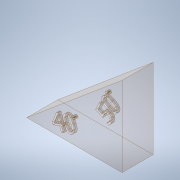
# Autodesk Inventor part: 40-50-4in-Template
Saved by Autodesk Inventor 2020.2 (Build 242310000, 310)
## iProperties
Created: 2020-01-27
Part Number: 40-50-4in-Template
Material: PET Plastic
Document SubType Name: Modeling
Designer: robst
Density: 1.541 g/cm^3
Appearance: Polycarbonate - Smoked
Author: robst
Autodesk Inventor part; units mm, degrees
ref_plane "YZ Plane" through (0, 0, 0) normal (1, 0, 0) x (0, 1, 0)
ref_plane "XZ Plane" through (0, 0, 0) normal (0, 1, 0) x (-1, 0, 0)
ref_plane "XY Plane" through (0, 0, 0) normal (0, 0, 1) x (1, 0, 0)
sketch "Sketch1" plane through (0, 0, 0) normal (0, 0, 1) x (1, 0, 0)
  line L0 (0, 0) -> (77.8301, 65.3072)
  line L1 (0, 0) -> (101.6, 0) construction
  line L2 (77.8301, 65.3072) -> (77.8301, 0)
  line L3 (77.8301, 0) -> (0, 0)
  dimension "d0" = 101.6
  dimension "d1" = 40
  constraints: 8 end point, 1 equal length, 1 horizontal, 1 perpendicular, 1 vertical
  measures "d0" distance of L0.start L0.end
  measures "d1" angle of L1 L0
extrude "Extrusion1" add sketch "Sketch1" along normal mid plane 25.4
sketch "Sketch2" plane through (0, 0, 12.7) normal (0, 0, 1) x (1, 0, 0)
  line L0 (0, 0) -> (77.8301, 0) construction
  line L1 (0, 0) -> (77.8301, 28.3278) construction
  line L2 (77.8301, 0) -> (77.8301, 65.3072) construction
  line L3 (29.7312, 8.7075) -> (28.3096, 8.1901)
  line L4 (28.3096, 8.1901) -> (29.8021, 4.0895)
  line L5 (29.8021, 4.0895) -> (28.2644, 3.5299)
  line L6 (28.2644, 3.5299) -> (26.7719, 7.6304)
  line L7 (26.7719, 7.6304) -> (21.5012, 5.712)
  line L8 (21.5012, 5.712) -> (20.8887, 7.3948)
  line L9 (20.8887, 7.3948) -> (23.9884, 15.4886)
  line L10 (23.9884, 15.4886) -> (25.4584, 16.0236)
  line L11 (25.4584, 16.0236) -> (27.8414, 9.4763)
  line L12 (27.8414, 9.4763) -> (29.2631, 9.9938)
  line L13 (29.2631, 9.9938) -> (29.7312, 8.7075)
  line L14 (26.3037, 8.9166) -> (24.6071, 13.5781)
  line L15 (24.6071, 13.5781) -> (22.2902, 7.4559)
  line L16 (22.2902, 7.4559) -> (26.3037, 8.9166)
  spline S0 degree 2 poles (37.7558, 13.742) (38.9245, 10.5312) (38.1527, 6.8442) (36.2088, 6.1366) knots 0 0 0 1 2 2 2
  spline S1 degree 2 poles (36.2088, 6.1366) (34.2359, 5.4186) (31.2729, 7.812) (30.1289, 10.9551) knots 0 0 0 1 2 2 2
  spline S2 degree 2 poles (30.1289, 10.9551) (28.9532, 14.1852) (29.7321, 17.8529) (31.6856, 18.564) knots 0 0 0 1 2 2 2
  spline S3 degree 2 poles (31.6856, 18.564) (33.6488, 19.2785) (36.6224, 16.8561) (37.7558, 13.742) knots 0 0 0 1 2 2 2
  spline S4 degree 2 poles (37.0291, 9.3594) (37.0465, 10.0339) (36.5781, 11.9224) (36.1311, 13.1506) knots 0 0 0 1 2 2 2
  spline S5 degree 2 poles (36.1311, 13.1506) (35.6841, 14.3789) (34.8324, 16.117) (34.3689, 16.6382) knots 0 0 0 1 2 2 2
  spline S6 degree 2 poles (34.3689, 16.6382) (33.9053, 17.1595) (32.8352, 17.4819) (32.1679, 17.239) knots 0 0 0 1 2 2 2
  spline S7 degree 2 poles (32.1679, 17.239) (31.5005, 16.9961) (30.8686, 16.0542) (30.846, 15.3341) knots 0 0 0 1 2 2 2
  spline S8 degree 2 poles (30.846, 15.3341) (30.826, 14.6368) (31.3277, 12.7166) (31.7536, 11.5464) knots 0 0 0 1 2 2 2
  spline S9 degree 2 poles (31.7536, 11.5464) (32.2112, 10.2892) (32.9784, 8.6627) (33.4692, 8.0966) knots 0 0 0 1 2 2 2
  spline S10 degree 2 poles (33.4692, 8.0966) (33.9266, 7.5622) (35.0302, 7.2081) (35.7266, 7.4616) knots 0 0 0 1 2 2 2
  spline S11 degree 2 poles (35.7266, 7.4616) (36.3842, 7.7009) (37.0161, 8.6428) (37.0291, 9.3594) knots 0 0 0 1 2 2 2
  spline S12 degree 2 poles (38.4763, 17.6439) (37.9694, 17.4594) (36.9953, 17.9137) (36.815, 18.409) knots 0 0 0 1 2 2 2
  spline S13 degree 2 poles (36.815, 18.409) (36.6305, 18.9159) (37.0848, 19.89) (37.5916, 20.0745) knots 0 0 0 1 2 2 2
  spline S14 degree 2 poles (37.5916, 20.0745) (38.087, 20.2548) (39.0611, 19.8005) (39.2456, 19.2937) knots 0 0 0 1 2 2 2
  spline S15 degree 2 poles (39.2456, 19.2937) (39.4259, 18.7983) (38.9716, 17.8242) (38.4763, 17.6439) knots 0 0 0 1 2 2 2
  spline S16 degree 2 poles (37.9564, 19.0723) (37.7375, 18.9926) (37.8172, 18.7738) knots 0 0 0 1 1 1
  spline S17 degree 2 poles (37.8172, 18.7738) (37.8926, 18.5664) (38.1115, 18.6461) knots 0 0 0 1 1 1
  spline S18 degree 2 poles (38.1115, 18.6461) (38.3189, 18.7216) (38.2434, 18.9289) knots 0 0 0 1 1 1
  spline S19 degree 2 poles (38.2434, 18.9289) (38.1637, 19.1478) (37.9564, 19.0723) knots 0 0 0 1 1 1
  dimension "d4" = 20
  constraints: 2 end point, 1 point on line, 1 other
  measures "d4" angle of L1 L0
sketch "Sketch3" plane through (0, 0, 12.7) normal (0, 0, 1) x (1, 0, 0)
  line L0 (77.8301, 65.3072) -> (0, 0) construction
  line L1 (77.8301, 65.3072) -> (47.3769, 0) construction
  line L2 (0, 0) -> (77.8301, 0) construction
  line L3 (77.8301, 0) -> (77.8301, 65.3072) construction
  spline S0 degree 2 poles (66.9517, 36.4992) (67.7819, 36.1121) (68.9517, 34.9193) (69.2479, 34.1907) knots 0 0 0 1 2 2 2
  spline S1 degree 2 poles (69.2479, 34.1907) (69.5441, 33.4621) (69.4762, 31.7336) (69.0586, 30.8382) knots 0 0 0 1 2 2 2
  spline S2 degree 2 poles (69.0586, 30.8382) (68.6759, 30.0174) (67.564, 28.5827) (67.0008, 28.1299) knots 0 0 0 1 2 2 2
  line L4 (67.0008, 28.1299) -> (65.3685, 28.891)
  line L5 (65.3685, 28.891) -> (65.4207, 29.003)
  spline S3 degree 2 poles (65.4207, 29.003) (65.6339, 29.1193) (66.2785, 29.625) (66.6148, 29.9564) knots 0 0 0 1 2 2 2
  spline S4 degree 2 poles (66.6148, 29.9564) (66.9865, 30.3395) (67.516, 31.0124) (67.7379, 31.4881) knots 0 0 0 1 2 2 2
  spline S5 degree 2 poles (67.7379, 31.4881) (67.9553, 31.9545) (68.0284, 32.9879) (67.8125, 33.4746) knots 0 0 0 1 2 2 2
  spline S6 degree 2 poles (67.8125, 33.4746) (67.6022, 33.9247) (66.8273, 34.6494) (66.2117, 34.9365) knots 0 0 0 1 2 2 2
  spline S7 degree 2 poles (66.2117, 34.9365) (65.5961, 35.2236) (64.656, 35.2531) (64.2469, 35.0578) knots 0 0 0 1 2 2 2
  spline S8 degree 2 poles (64.2469, 35.0578) (63.8056, 34.8662) (63.1107, 34.0092) (62.8367, 33.4216) knots 0 0 0 1 2 2 2
  spline S9 degree 2 poles (62.8367, 33.4216) (62.5409, 32.7873) (62.1496, 31.4367) (62.0552, 31.0152) knots 0 0 0 1 2 2 2
  line L6 (62.0552, 31.0152) -> (56.123, 33.7814)
  line L7 (56.123, 33.7814) -> (59.0675, 40.0961)
  line L8 (59.0675, 40.0961) -> (60.42, 39.4655)
  line L9 (60.42, 39.4655) -> (58.167, 34.6338)
  line L10 (58.167, 34.6338) -> (61.2357, 33.2029)
  spline S10 degree 2 poles (61.2357, 33.2029) (61.3289, 33.5001) (61.5532, 34.0541) (61.6576, 34.278) knots 0 0 0 1 2 2 2
  spline S11 degree 2 poles (61.6576, 34.278) (62.0708, 35.1641) (62.9297, 36.2512) (63.6198, 36.6107) knots 0 0 0 1 2 2 2
  spline S12 degree 2 poles (63.6198, 36.6107) (64.3141, 36.9796) (65.9071, 36.9863) (66.9517, 36.4992) knots 0 0 0 1 2 2 2
  spline S13 degree 2 poles (68.9677, 46.3016) (72.0644, 44.8576) (74.1258, 41.7047) (73.2515, 39.8299) knots 0 0 0 1 2 2 2
  spline S14 degree 2 poles (73.2515, 39.8299) (72.3642, 37.9271) (68.5767, 37.5243) (65.5452, 38.9379) knots 0 0 0 1 2 2 2
  spline S15 degree 2 poles (65.5452, 38.9379) (62.4299, 40.3906) (60.3871, 43.5348) (61.2657, 45.4189) knots 0 0 0 1 2 2 2
  spline S16 degree 2 poles (61.2657, 45.4189) (62.1487, 47.3124) (65.9642, 47.7021) (68.9677, 46.3016) knots 0 0 0 1 2 2 2
  spline S17 degree 2 poles (71.5527, 42.6888) (71.0881, 43.178) (69.4215, 44.1822) (68.2369, 44.7346) knots 0 0 0 1 2 2 2
  spline S18 degree 2 poles (68.2369, 44.7346) (67.0523, 45.287) (65.2211, 45.9138) (64.5248, 45.9546) knots 0 0 0 1 2 2 2
  spline S19 degree 2 poles (64.5248, 45.9546) (63.8284, 45.9954) (62.8437, 45.4667) (62.5436, 44.8231) knots 0 0 0 1 2 2 2
  spline S20 degree 2 poles (62.5436, 44.8231) (62.2435, 44.1795) (62.4626, 43.0666) (62.9558, 42.5414) knots 0 0 0 1 2 2 2
  spline S21 degree 2 poles (62.9558, 42.5414) (63.4347, 42.0342) (65.1473, 41.0312) (66.276, 40.5049) knots 0 0 0 1 2 2 2
  spline S22 degree 2 poles (66.276, 40.5049) (67.4885, 39.9395) (69.1811, 39.3319) (69.9285, 39.2786) knots 0 0 0 1 2 2 2
  spline S23 degree 2 poles (69.9285, 39.2786) (70.6298, 39.2241) (71.6605, 39.7542) (71.9737, 40.4257) knots 0 0 0 1 2 2 2
  spline S24 degree 2 poles (71.9737, 40.4257) (72.2694, 41.06) (72.0502, 42.1729) (71.5527, 42.6888) knots 0 0 0 1 2 2 2
  spline S25 degree 2 poles (66.718, 49.5701) (66.4901, 49.0812) (65.48, 48.7136) (65.0023, 48.9364) knots 0 0 0 1 2 2 2
  spline S26 degree 2 poles (65.0023, 48.9364) (64.5135, 49.1643) (64.1458, 50.1744) (64.3738, 50.6632) knots 0 0 0 1 2 2 2
  spline S27 degree 2 poles (64.3738, 50.6632) (64.5966, 51.141) (65.6066, 51.5086) (66.0954, 51.2806) knots 0 0 0 1 2 2 2
  spline S28 degree 2 poles (66.0954, 51.2806) (66.5732, 51.0579) (66.9408, 50.0478) (66.718, 49.5701) knots 0 0 0 1 2 2 2
  spline S29 degree 2 poles (65.3404, 50.2125) (65.2419, 50.0014) (65.453, 49.903) knots 0 0 0 1 1 1
  spline S30 degree 2 poles (65.453, 49.903) (65.653, 49.8097) (65.7514, 50.0208) knots 0 0 0 1 1 1
  spline S31 degree 2 poles (65.7514, 50.0208) (65.8447, 50.2208) (65.6447, 50.314) knots 0 0 0 1 1 1
  spline S32 degree 2 poles (65.6447, 50.314) (65.4336, 50.4125) (65.3404, 50.2125) knots 0 0 0 1 1 1
  dimension "d5" = 25
  constraints: 2 end point, 1 point on line, 1 other
  measures "d5" angle of L1 L3
extrude "Extrusion2" cut sketch "Sketch2" against normal blind 2.54
extrude "Extrusion3" cut sketch "Sketch3" against normal blind 2.54
body "Solid1"
